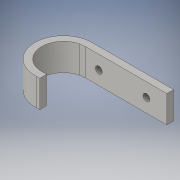
# Autodesk Inventor part: Brazo
Saved by Autodesk Inventor 2016 (Build 200138000, 138)
## iProperties
Created: 2016-02-20
Part Number: Brazo
Material: Generic
Document SubType Name: Modeling
Designer: Admin
Density: 1 g/cm^3
Appearance: Default
Author: Admin
Autodesk Inventor part; units mm, degrees
ref_plane "YZ Plane" through (0, 0, 0) normal (1, 0, 0) x (0, 1, 0)
ref_plane "XZ Plane" through (0, 0, 0) normal (0, 1, 0) x (-1, 0, 0)
ref_plane "XY Plane" through (0, 0, 0) normal (0, 0, 1) x (1, 0, 0)
sketch "Sketch1" plane through (0, 0, 0) normal (0, 1, 0) x (-1, 0, 0)
  line L0 (21.8478, -20.797) -> (-54.3522, -20.797)
  line L1 (-54.3522, -20.797) -> (-54.3522, -14.447)
  line L2 (-54.3522, -14.447) -> (21.8478, -14.447)
  line L3 (21.8478, -20.797) -> (6.1545, 27.502) construction
  line L4 (21.8478, -20.797) -> (72.6323, -20.797) construction
  arc A0 (26.301, -13.9537) -> (20.5574, 26.2101) centre (21.8478, 5.9021) ccw
  line L5 (26.301, -13.9537) -> (26.2938, -13.9315)
  line L6 (26.2938, -13.9315) -> (21.8478, -14.447)
  line L7 (20.5574, 26.2101) -> (17.3824, 26.2101)
  arc A1 (21.8478, -20.797) -> (20.5574, 32.5699) centre (21.8478, 5.9021) ccw
  line L8 (20.5574, 32.5699) -> (17.3824, 32.5699)
  line L9 (17.3824, 32.5699) -> (17.3824, 26.2101)
  point P0 (0, 0)
  dimension "d5" = 6.35
  dimension "d6" = 76.2
  dimension "d7" = 76.2
  dimension "d10" = 50.7846
  dimension "d11" = 108
  dimension "d13" = 3.175
  constraints: 20 end point, 4 point on circle, 3 horizontal, 3 perpendicular, 2 centre point, 1 equal length, 1 tangent
  measures "d5" distance of L0.end L1.end
  measures "d6" distance of L1.end L2.end
  measures "d7" distance of L0.start L0.end
  measures "d10" distance of L0.start L3.end
  measures "d11" angle of L4 L3
  measures "d13" distance of L7.start L7.end
extrude "Extrusion1" add sketch "Sketch1" along normal blind 25.4
sketch "Sketch2" plane through (-21.8478, 0, -14.447) normal (0, 0, 1) x (1, 0, 0)
  circle A0 centre (57.15, 12.7) radius 3.175
  circle A1 centre (12.7, 12.7) radius 3.175
  line L0 (76.2, 0) -> (76.2, 25.4) projected
  point P0 (21.8478, 0)
  dimension "d17" = 6.35
  dimension "d18" = 6.35
  dimension "d19" = 19.05
  dimension "d20" = 63.5
  constraints: 2 centre point
  measures "d17" diameter of A0
  measures "d18" diameter of A1
  measures "d19" distance from line of L0 A0.centre
  measures "d20" distance from line of L0 A1.centre
extrude "Extrusion2" cut sketch "Sketch2" against normal blind 6.35
body "Solid1"
